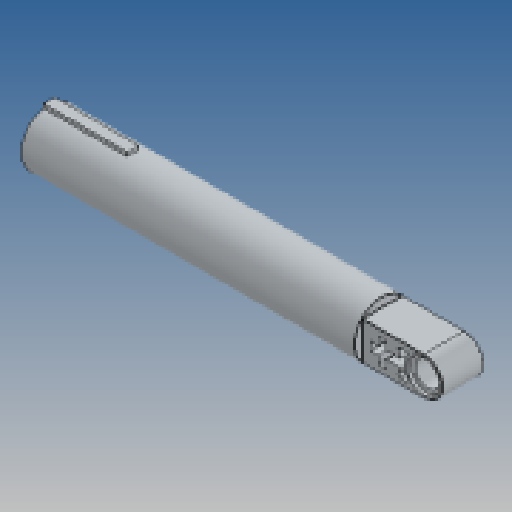
# Autodesk Inventor part: 67498_02
Saved by Autodesk Inventor 2025 (Build 290162010, 162A)
## iProperties
Created: 2024-12-01
Part Number: 67498_02
Material: ABS-Kunststoff
Document SubType Name: Modeling
Designer: hp.muther
Density: 1.06 g/cm^3
Appearance: LtBluishGray
Author: hp.muther
Autodesk Inventor part; units mm, degrees
ref_plane "YZ Plane" through (0, 0, 0) normal (1, 0, 0) x (0, 1, 0)
ref_plane "XZ Plane" through (0, 0, 0) normal (0, 1, 0) x (-1, 0, 0)
ref_plane "XY Plane" through (0, 0, 0) normal (0, 0, 1) x (1, 0, 0)
sketch "Skizze1" plane through (0, 0, 0) normal (0, 1, 0) x (-1, 0, 0)
  line L0 (0, 0) -> (-65, 0)
  line L1 (0, 0) -> (0, 5.45)
  line L2 (0, 5.45) -> (-65, 5.45)
  line L3 (-65, 5.45) -> (-65, 0)
  line L4 (0, 4.4) -> (-63, 4.4)
  line L5 (-63, 4.4) -> (-63, 0)
  dimension "d0" = 65
  dimension "d1" = 10.9
  dimension "d2" = 63
  dimension "d3" = 8.8
  constraints: 12 end point, 3 perpendicular, 2 horizontal, 2 point on line, 1 vertical
  measures "d0" distance of L0.start L0.end
  measures "d1" diameter of L2 L0
  measures "d2" distance of L4.start L4.end
  measures "d3" diameter of L4 L0
revolve "Umdrehung1" add sketch "Skizze1" angle 360 about axis through (0, 0, 0) along (1, 0, 0) contours L0 L3 L2 L1 L4 L5
sketch "Skizze2" plane through (0, 0, 0) normal (-1, 0, 0) x (0, 0, 1)
  circle A0 centre (0, 0) radius 5.45 projected
  line L0 (6.1, 1.1) -> (-6.1, 1.1)
  line L1 (-6.1, 1.1) -> (-6.1, -1.1)
  line L2 (-6.1, -1.1) -> (6.1, -1.1)
  line L3 (6.1, -1.1) -> (6.1, 1.1)
  point P0 (0, 1.1)
  point P1 (-6.1, 0)
  point P2 (5.3378, 1.1)
  point P3 (5.3378, -1.1)
  point P4 (-5.3378, -1.1)
  point P5 (-5.3378, 1.1)
  dimension "d5" = 2.2
  dimension "d6" = 12.2
  constraints: 8 end point, 2 midpoint, 2 parallel, 1 horizontal, 1 horizontal alignment, 1 perpendicular, 1 vertical alignment
  measures "d5" distance between parallel lines of L2 L0
  measures "d6" distance of L0.start L0.end
extrude "Extrusion1" add sketch "Skizze2" against normal blind 16.4 contours A0 L0 L3 L2 | A0 L2 L1 L0
sketch "Skizze3" plane through (0, 0, 0) normal (0, 1, 0) x (-1, 0, 0)
  line L0 (-65, -3.7) -> (-65, 3.7)
  line L1 (-65, 3.7) -> (-77, 3.7)
  arc A0 (-77, 3.7) -> (-77, -3.7) centre (-77, 0) ccw
  line L2 (-77, -3.7) -> (-65, -3.7)
  circle A1 centre (-77, 0) radius 2.4
  line L3 (-65, 5.45) -> (-65, -5.45) projected
  circle A2 centre (-69, 0) radius 2.4
  arc A3 (-73.8778, -1.9854) -> (-73.8778, 1.9854) centre (-77, 0) ccw
  line L4 (-73.5402, 2.6) -> (-72.4598, 2.6)
  line L5 (-73.5402, -2.6) -> (-72.4598, -2.6)
  arc A4 (-72.1222, 1.9854) -> (-72.1222, -1.9854) centre (-69, 0) ccw
  arc A5 (-73.5402, 2.6) -> (-73.8778, 1.9854) centre (-73.5402, 2.2) ccw
  arc A6 (-72.1222, 1.9854) -> (-72.4598, 2.6) centre (-72.4598, 2.2) ccw
  arc A7 (-72.4598, -2.6) -> (-72.1222, -1.9854) centre (-72.4598, -2.2) ccw
  arc A8 (-73.8778, -1.9854) -> (-73.5402, -2.6) centre (-73.5402, -2.2) ccw
  line L6 (-69.8, 2.2627) -> (-69.8, 0.8)
  line L7 (-69.8, 0.8) -> (-72.6125, 0.8)
  line L8 (-72.6125, -0.8) -> (-69.8, -0.8)
  line L9 (-69.8, -0.8) -> (-69.8, -2.2627)
  line L10 (-68.2, -0.8) -> (-66.7373, -0.8)
  line L11 (-68.2, 0.8) -> (-66.7373, 0.8)
  line L12 (-68.2, 0.8) -> (-68.2, 2.2627)
  line L13 (-68.2, -0.8) -> (-68.2, -2.2627)
  point P0 (0, 0)
  point P1 (-65, 0)
  point P2 (-74.0537, -2.2382)
  point P3 (-74.3675, 2.6)
  point P4 (-71.6325, 2.6)
  point P5 (-74.3675, -2.6)
  point P6 (-71.6325, -2.6)
  dimension "d9" = 7.4
  dimension "d10" = 12
  dimension "d11" = 4.8
  dimension "d12" = 0.4
  dimension "d13" = 1.1
  dimension "d14" = 8
  dimension "d15" = 1.6
  constraints: 27 point on circle, 26 end point, 10 point on line, 10 tangent, 9 centre point, 7 equal length, 6 equal radius, 3 perpendicular, 2 concentric, 2 horizontal, 2 midpoint, 2 vertical, 1 coincident, 1 collinear, 1 horizontal alignment
  measures "d9" distance between parallel lines of L2 L1
  measures "d10" distance from line of A0.centre L0
  measures "d11" diameter of A1
  measures "d12" radius of A5
  measures "d13" distance between parallel lines of L1 L4
  measures "d14" distance of A1.centre A2.centre
  measures "d15" distance between parallel lines of L10 L11
extrude "Extrusion2" add sketch "Skizze3" along normal mid plane 8 contours L2 A0 L1 L0 | L11 L12 A2 | A2 L13 L10 | L6 L7 A2 | A2 L8 L9
sketch "Skizze4" plane through (0, -4, 0) normal (0, -1, 0) x (1, 0, 0)
  circle A0 centre (77, 0) radius 2.4 projected
  circle A1 centre (77, 0) radius 3.2
  point P0 (0, 0)
  dimension "d18" = 6.4
  constraints: 1 centre point, 1 coincident
  measures "d18" diameter of A1
extrude "Extrusion3" cut sketch "Skizze4" against normal blind 0.8
sketch "Skizze5" plane through (0, 4, 0) normal (0, 1, 0) x (1, 0, 0)
  circle A0 centre (77, 0) radius 2.4 projected
  circle A1 centre (77, 0) radius 3.2 projected
  point P0 (0, 0)
extrude "Extrusion4" cut sketch "Skizze5" against normal blind 0.8
sketch "Skizze6" plane through (0, 4, 0) normal (0, 1, 0) x (1, 0, 0)
  arc A0 (72.4598, 2.6) -> (72.1222, 1.9854) centre (72.4598, 2.2) ccw projected
  arc A1 (72.1222, -1.9854) -> (72.4598, -2.6) centre (72.4598, -2.2) ccw projected
  arc A2 (72.1222, -1.9854) -> (72.6125, -0.8) centre (69, 0) ccw projected
  line L0 (72.6125, -0.8) -> (69.8, -0.8) projected
  line L1 (69.8, -0.8) -> (69.8, -2.2627) projected
  line L2 (69.8, 2.2627) -> (69.8, 0.8) projected
  line L3 (69.8, 0.8) -> (72.6125, 0.8) projected
  arc A3 (72.6125, 0.8) -> (72.1222, 1.9854) centre (69, 0) ccw projected
  line L4 (69.8, 1.6) -> (72.0598, 1.6)
  line L5 (72.0598, -1.6) -> (69.8, -1.6)
  line L6 (69.8, -1.6) -> (69.8, 1.6)
  line L7 (72.6125, 0.8) -> (69.8, 0.8) projected
  line L8 (72.0598, 2.2) -> (72.0598, 1.6)
  line L9 (72.0598, -1.6) -> (72.0598, -2.2)
  point P0 (0, 0)
  point P1 (69.8, 0)
  dimension "d23" = 2.4
  constraints: 10 end point, 2 collinear, 2 point on circle, 2 tangent, 1 horizontal, 1 horizontal alignment, 1 midpoint, 1 parallel, 1 point on line
  measures "d23" distance between parallel lines of L7 L5
extrude "Extrusion5" cut sketch "Skizze6" against normal blind 0.3
sketch "Skizze7" plane through (0, 3.7, 0) normal (0, 1, 0) x (1, 0, 0)
  arc A0 (72.0598, 2.2) -> (72.1222, 1.9854) centre (72.4598, 2.2) ccw projected
  line L0 (72.6125, 0.8) -> (69.8, 0.8) projected
  arc A1 (72.6125, 0.8) -> (72.1222, 1.9854) centre (69, 0) ccw projected
  line L1 (72.0598, -2.2) -> (72.0598, -1.6) projected
  line L2 (72.0598, -1.6) -> (69.8, -1.6) projected
  line L3 (69.8, -1.6) -> (69.8, -2.2627) projected
  arc A2 (68.2, -2.2627) -> (69.8, -2.2627) centre (69, 0) ccw projected
  line L4 (68.2, -2.2627) -> (68.2, -0.8) projected
  line L5 (68.2, -0.8) -> (66.7373, -0.8) projected
  arc A3 (66.7373, 0.8) -> (66.7373, -0.8) centre (69, 0) ccw projected
  line L6 (66.7373, 0.8) -> (68.2, 0.8) projected
  line L7 (68.2, 0.8) -> (68.2, 2.2627) projected
  arc A4 (69.8, 2.2627) -> (68.2, 2.2627) centre (69, 0) ccw projected
  line L8 (69.8, 2.2627) -> (69.8, 1.6) projected
  line L9 (69.8, 1.6) -> (72.0598, 1.6) projected
  line L10 (72.0598, 1.6) -> (72.0598, 2.2) projected
  arc A5 (72.4598, 2.6) -> (72.0598, 2.2) centre (72.4598, 2.2) ccw projected
  line L11 (72.4598, 2.6) -> (73.5402, 2.6) projected
  arc A6 (73.8778, 1.9854) -> (73.5402, 2.6) centre (73.5402, 2.2) ccw projected
  arc A7 (73.8778, 1.9854) -> (73.8778, -1.9854) centre (77, 0) ccw projected
  arc A8 (73.5402, -2.6) -> (73.8778, -1.9854) centre (73.5402, -2.2) ccw projected
  line L12 (73.5402, -2.6) -> (72.4598, -2.6) projected
  arc A9 (72.0598, -2.2) -> (72.4598, -2.6) centre (72.4598, -2.2) ccw projected
  line L13 (77, 3.7) -> (65, 3.7) projected
  line L14 (65, -3.7) -> (65, 3.7) projected
  line L15 (65, -3.7) -> (77, -3.7) projected
  arc A10 (77, -3.7) -> (77, 3.7) centre (77, 0) ccw projected
  circle A11 centre (77, 0) radius 3.2 projected
  line L16 (69.8, -0.8) -> (72.6125, -0.8) projected
  line L17 (69.8, -1.6) -> (69.8, -0.8) projected
  line L18 (72.0598, -1.6) -> (69.8, -1.6) projected
  line L19 (72.0598, -2.2) -> (72.0598, -1.6) projected
  arc A12 (72.1222, -1.9854) -> (72.0598, -2.2) centre (72.4598, -2.2) ccw projected
  arc A13 (72.1222, -1.9854) -> (72.6125, -0.8) centre (69, 0) ccw projected
  arc A14 (71.2627, -0.8) -> (71.2627, 0.8) centre (69, 0) ccw
  point P0 (0, 0)
  constraints: 2 concentric, 2 point on circle, 2 point on line, 1 centre point
extrude "Extrusion6" add sketch "Skizze7" against normal blind 0.8 contours A5 L11 A6 A7 A8 L12 A9 A12 A13 L16 A14 L0 A1 A0
fillet "Rundung1" radius 0.1 7 edges at (80.7, 4, 0) (71, 4, -3.7) (71, 4, 3.7) (80.7, -4, 0) (71, -4, -3.7) (71, -4, 3.7) (65, 0, -5.45)
fillet "Rundung2" radius 0.1 16 edges at (64.9987, -4, 3.5768) (64.9819, -3.97, 3.6714) (64.9991, -3.8823, 3.7) (65, 0, 3.7) (64.9991, 3.8823, 3.7) (64.9819, 3.97, 3.6714) (64.9987, 4, 3.5768) (65, 4, 0) (64.9987, 4, -3.5768) (64.9819, 3.97, -3.6714) (64.9991, 3.8823, -3.7) (65, 0, -3.7) (64.9991, -3.8823, -3.7) (64.9819, -3.97, -3.6714) (64.9987, -4, -3.5768) (65, -4, 0)
